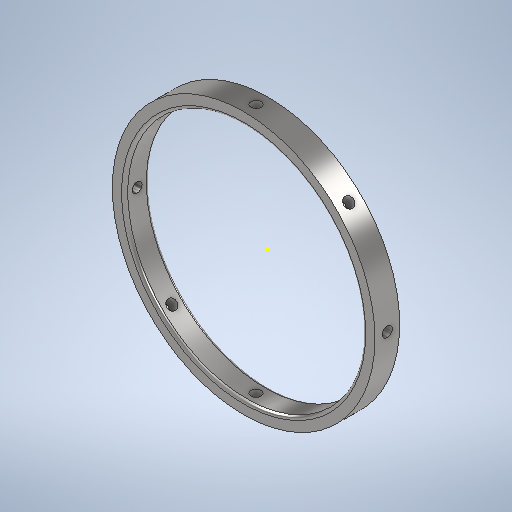
# Autodesk Inventor part: Flywheel inner ring
Saved by Autodesk Inventor 2025.2 (Build 292293000, 293)
## iProperties
Created: 2025-06-12
Part Number: Flywheel inner ring
Material: Steel, Carbon
Document SubType Name: Modeling
Designer: bless
Density: 7.85 g/cm^3
Appearance: Semi-Polished
Author: bless
Autodesk Inventor part; units mm, degrees
ref_plane "XZ Plane" through (0, 0, 0) normal (0, 1, 0) x (-1, 0, 0)
ref_plane "XY Plane" through (0, 0, 0) normal (0, 0, 1) x (1, 0, 0)
sketch "Sketch1" plane through (0, 0, 0) normal (0, 0, 1) x (1, 0, 0)
  circle A0 centre (0, 0) radius 85
  circle A1 centre (0, 0) radius 77
  dimension "d0" = 170
  dimension "d1" = 154
  constraints: 2 centre point, 2 coincident
  measures "d0" diameter of A0
  measures "d1" diameter of A1
extrude "Extrusion1" add sketch "Sketch1" along normal blind 16
fillet "Fillet1" radius 2 2 edges at (-77, 0, 16) (-77, 0, 0)
sketch "Sketch2" plane through (0, 0, 0) normal (1, 0, 0) x (0, 1, 0)
  point P0 (0, 0)
ref_plane "Work Plane1" through (85, 0, 0) normal (1, 0, 0) x (0, 1, 0)
sketch "Sketch3" plane through (85, 0, 0) normal (1, 0, 0) x (0, 1, 0)
  circle A0 centre (0, 8) radius 3.25
  point P0 (0, 0)
  dimension "d6" = 6.5
  dimension "d7" = 8
  constraints: 1 centre point, 1 vertical alignment
  measures "d6" diameter of A0
  measures "d7" distance of A0.centre point (0, 0)
extrude "Extrusion2" cut sketch "Sketch3" against normal up to surface
pattern_circular "Circular Pattern1" count 8 over 360 about axis through (0, 0, 14) along (0, 0, -1) of "Extrusion2"
body "Solid1"
